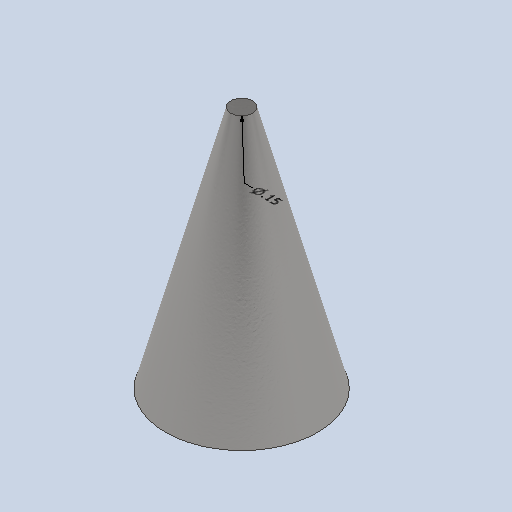
# Autodesk Inventor part: CC-01
Saved by Autodesk Inventor 2022 (Build 260153000, 153)
## iProperties
Company: El Camino College
Created: 2023-06-01
Part Number: CC-01
Material: Steel, Galvanized
Document SubType Name: Modeling
Designer: Edgar Tejada
Density: 7.85 g/cm^3
Appearance: Galvanized
Mass: 11.9178 g
Surface Area: 39.1531 cm^2
Volume: 1.51819 cm^3
Description: Steel Collet Cone
Author: Edgar Tejada
Title: Collet Cone
Autodesk Inventor part; units mm, degrees
ref_plane "YZ Plane" through (0, 0, 0) normal (1, 0, 0) x (0, 1, 0)
ref_plane "XZ Plane" through (0, 0, 0) normal (0, 1, 0) x (-1, 0, 0)
ref_plane "XY Plane" through (0, 0, 0) normal (0, 0, 1) x (1, 0, 0)
sketch "Sketch1" plane through (0, 0, 0) normal (0, 0, 1) x (1, 0, 0)
  line L0 (0, 0) -> (0, 41.4782)
  line L1 (0, 41.4782) -> (-1.27, 41.4782)
  line L2 (-1.27, 41.4782) -> (-12.3841, 0)
  line L3 (-12.3841, 0) -> (0, 0)
  line L4 (0, -8.2956) -> (0, 49.7738) projected
  dimension "d0" = 1.27
  dimension "d1" = 75
  dimension "d2" = 41.4782
  constraints: 8 end point, 1 parallel, 1 perpendicular, 1 vertical
  measures "d0" distance of L0.end L1.end
  measures "d1" angle of L3 L2
  measures "d2" distance of L0.start L0.end
revolve "Revolution1" add sketch "Sketch1" angle 360 about axis through (0, -10, 0) along (0, 1, 0)
shell "Shell1" thickness 0.7937 outward yes removed faces 1 at (4.0081, 0, 0.9879)
sketch "Sketch2" plane through (0, 0, 0) normal (1, 0, 0) x (0, 1, 0)
  line L0 (0, 0) -> (12.7, 0) construction
  line L1 (0, -1.7996) -> (12.7, -1.7996)
  line L2 (12.7, 1.7996) -> (0, 1.7996)
  arc A0 (0, 1.7996) -> (0, -1.7996) centre (0, 0) ccw
  arc A1 (12.7, -1.7996) -> (12.7, 1.7996) centre (12.7, 0) ccw
  line L3 (0, -13.2058) -> (0, 13.2058) projected
  point P0 (6.35, 0)
  dimension "d7" = 1.7996
  dimension "d8" = 6.35
  constraints: 8 end point, 4 point on circle, 4 tangent, 2 centre point, 1 horizontal, 1 midpoint, 1 parallel
  measures "d7" radius of A0
  measures "d8" distance from line of point (6.35, 0) L3
extrude "Extrusion1" cut sketch "Sketch2" against normal through all contours L3 L2 A1 L1
body "Solid1"
